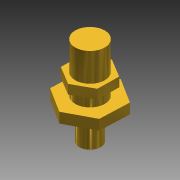
# Autodesk Inventor part: SMA_Bulkhead
Saved by Autodesk Inventor 2014 (Build 180170000, 170)
## iProperties
Created: 2015-03-25
Part Number: SMA_Bulkhead
Material: Generic
Document SubType Name: Modeling
Designer: Owner
Density: 1 g/cm^3
Appearance: Gold - Metal
Author: Owner
Autodesk Inventor part; units mm, degrees
ref_plane "YZ Plane" through (0, 0, 0) normal (1, 0, 0) x (0, 1, 0)
ref_plane "XZ Plane" through (0, 0, 0) normal (0, 1, 0) x (-1, 0, 0)
ref_plane "XY Plane" through (0, 0, 0) normal (0, 0, 1) x (1, 0, 0)
sketch "Sketch1" plane through (0, 0, 0) normal (0, 1, 0) x (-1, 0, 0)
  circle A0 centre (0, 0) radius 2.3
  dimension "d0" = 4.6
  constraints: 1 centre point, 1 coincident
  measures "d0" diameter of A0
extrude "Extrusion1" add sketch "Sketch1" along normal blind 6.3
sketch "Sketch2" plane through (0, 6.3, 0) normal (0, 1, 0) x (1, 0, 0)
  circle A0 centre (0, 0) radius 2.3 projected
  line L0 (5.6221, 2.954) -> (5.3692, -3.3919)
  line L1 (5.3692, -3.3919) -> (-0.2528, -6.3458)
  line L2 (-0.2528, -6.3458) -> (-5.6221, -2.954)
  line L3 (-5.6221, -2.954) -> (-5.3692, 3.3919)
  line L4 (-5.3692, 3.3919) -> (0.2528, 6.3458)
  line L5 (0.2528, 6.3458) -> (5.6221, 2.954)
  dimension "d10" = 11
  constraints: 12 end point, 1 coincident, 13 other
  measures "d10" distance between parallel lines of L2 L5
extrude "Extrusion2" add sketch "Sketch2" along normal blind 2.2 contours A0 | L0 L1 L2 L3 L4 L5
sketch "Sketch3" plane through (0, 8.5, 0) normal (0, 1, 0) x (1, 0, 0)
  circle A0 centre (0, 0) radius 3.175
  dimension "d6" = 6.35
  constraints: 1 centre point, 1 coincident
  measures "d6" diameter of A0
extrude "Extrusion3" add sketch "Sketch3" along normal blind 2.4
sketch "Sketch4" plane through (0, 10.9, 0) normal (0, 1, 0) x (1, 0, 0)
  circle A0 centre (0, 0) radius 3.175 projected
  line L0 (4.0415, 2.236) -> (3.9572, -2.3821)
  line L1 (3.9572, -2.3821) -> (-0.0844, -4.618)
  line L2 (-0.0844, -4.618) -> (-4.0415, -2.236)
  line L3 (-4.0415, -2.236) -> (-3.9572, 2.3821)
  line L4 (-3.9572, 2.3821) -> (0.0844, 4.618)
  line L5 (0.0844, 4.618) -> (4.0415, 2.236)
  dimension "d9" = 8
  constraints: 12 end point, 1 coincident, 13 other
  measures "d9" distance between parallel lines of L2 L5
extrude "Extrusion4" add sketch "Sketch4" along normal blind 2 contours A0 | L0 L1 L2 L3 L4 L5
sketch "Sketch5" plane through (0, 12.9, 0) normal (0, 1, 0) x (1, 0, 0)
  circle A0 centre (0, 0) radius 3.175
  dimension "d13" = 6.35
  constraints: 1 centre point, 1 coincident
  measures "d13" diameter of A0
extrude "Extrusion5" add sketch "Sketch5" along normal blind 6.1
body "Solid1"
